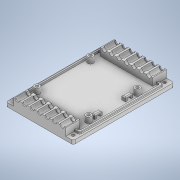
# Autodesk Inventor part: Enclosure Box
Saved by Autodesk Inventor 2021 (Build 250183000, 183)
## iProperties
Created: 2021-06-04
Part Number: Enclosure Box
Material: Generic
Document SubType Name: Modeling
Designer: Anton
Density: 1 g/cm^3
Appearance: Default
Author: Anton
Autodesk Inventor part; units mm, degrees
ref_plane "YZ Plane" through (0, 0, 0) normal (1, 0, 0) x (0, 1, 0)
ref_plane "XZ Plane" through (0, 0, 0) normal (0, 1, 0) x (-1, 0, 0)
ref_plane "XY Plane" through (0, 0, 0) normal (0, 0, 1) x (1, 0, 0)
sketch "Sketch2" plane through (0, 0, 0) normal (0, 1, 0) x (-1, 0, 0)
  line L0 (0, 0) -> (62, 0)
  line L1 (62, 0) -> (62, -66)
  line L2 (62, -66) -> (0, -66)
  line L3 (0, -66) -> (0, 0)
  circle A0 centre (58.15, -9.3) radius 1.5
  circle A1 centre (57.35, -60.86) radius 1.5
  circle A2 centre (3, -4.5) radius 1.5
  circle A3 centre (3, -61.9) radius 1.5
  circle A4 centre (3, -4.5) radius 3
  circle A5 centre (58.15, -9.3) radius 3
  circle A6 centre (57.35, -60.86) radius 3
  circle A7 centre (3, -61.9) radius 3
  line L4 (63, 20) -> (-1, 20)
  line L5 (-1, 20) -> (-1, -86)
  line L6 (-1, -86) -> (63, -86)
  line L7 (63, -86) -> (63, 20)
  dimension "d14" = 66
  dimension "d15" = 62
  dimension "d16" = 3
  dimension "d17" = 3
  dimension "d18" = 3
  dimension "d19" = 3
  dimension "d20" = 3
  dimension "d21" = 4.5
  dimension "d22" = 6
  dimension "d23" = 3
  dimension "d24" = 57.4
  dimension "d25" = 54.35
  dimension "d26" = 0.8
  dimension "d27" = 51.56
  dimension "d28" = 4.8
  dimension "d29" = 6
  dimension "d30" = 6
  dimension "d31" = 6
  dimension "d32" = 20
  dimension "d33" = 20
  dimension "d34" = 1
  dimension "d35" = 1
  constraints: 16 end point, 8 centre point, 4 coincident, 4 parallel, 2 horizontal, 2 perpendicular
  measures "d14" distance between parallel lines of L2 L0
  measures "d15" distance between parallel lines of L3 L1
  measures "d16" diameter of A0
  measures "d17" diameter of A1
  measures "d18" diameter of A3
  measures "d19" diameter of A2
  measures "d20" distance from line of L3 A2.centre
  measures "d21" distance from line of A2.centre L0
  measures "d22" diameter of A4
  measures "d23" distance from line of L3 A3.centre
  measures "d24" distance of A2.centre A3.centre
  measures "d25" horizontal distance of A1.centre A3.centre
  measures "d26" horizontal distance of A1.centre A0.centre
  measures "d27" vertical distance of A1.centre A0.centre
  measures "d28" vertical distance of A2.centre A0.centre
  measures "d29" diameter of A5
  measures "d30" diameter of A6
  measures "d31" diameter of A7
  measures "d32" distance between parallel lines of L4 L0
  measures "d33" distance between parallel lines of L2 L6
  measures "d34" distance between parallel lines of L7 L1
  measures "d35" distance between parallel lines of L3 L5
extrude "Extrusion1" add sketch "Sketch2" along normal blind 2 contours A4 | A7 | L0 L1 L2 L3 | A0 | A1 | A2 | A3 | A5 | A6 | L7 L6 L5 L4
sketch "Sketch4" plane through (0, 2, 0) normal (0, 1, 0) x (1, 0, 0)
  line L0 (-62, 66) -> (0, 66)
  line L1 (0, 66) -> (0, 0)
  line L2 (0, 0) -> (-62, 0)
  line L3 (-62, 0) -> (-62, 66)
  circle A0 centre (-3.85, 56.7) radius 1.5
  circle A1 centre (-4.65, 5.14) radius 1.5
  circle A2 centre (-59, 61.5) radius 1.5
  circle A3 centre (-59, 4.1) radius 1.5
  circle A4 centre (-59, 61.5) radius 3
  circle A5 centre (-3.85, 56.7) radius 3
  circle A6 centre (-4.65, 5.14) radius 3
  circle A7 centre (-59, 4.1) radius 3
  line L4 (1, 86) -> (-63, 86)
  line L5 (-63, 86) -> (-63, -20)
  line L6 (-63, -20) -> (1, -20)
  line L7 (1, -20) -> (1, 86)
  line L8 (1, 86) -> (-63, 86) projected
  line L9 (-63, 86) -> (-63, -20) projected
  point P0 (0, 0)
  dimension "d38" = 66
  dimension "d39" = 62
  dimension "d40" = 3
  dimension "d41" = 3
  dimension "d42" = 3
  dimension "d43" = 3
  dimension "d44" = 3
  dimension "d45" = 4.5
  dimension "d46" = 6
  dimension "d47" = 3
  dimension "d48" = 57.4
  dimension "d49" = 54.35
  dimension "d50" = 0.8
  dimension "d51" = 51.56
  dimension "d52" = 4.8
  dimension "d53" = 6
  dimension "d54" = 6
  dimension "d55" = 6
  dimension "d56" = 20
  dimension "d57" = 20
  dimension "d58" = 1
  dimension "d59" = 1
  dimension "d60" = 0
  dimension "d61" = 0
  constraints: 16 end point, 8 centre point, 4 coincident, 4 parallel, 2 horizontal, 2 perpendicular
  measures "d38" distance between parallel lines of L2 L0
  measures "d39" distance between parallel lines of L3 L1
  measures "d40" diameter of A0
  measures "d41" diameter of A1
  measures "d42" diameter of A3
  measures "d43" diameter of A2
  measures "d44" distance from line of L3 A2.centre
  measures "d45" distance from line of A2.centre L0
  measures "d46" diameter of A4
  measures "d47" distance from line of L3 A3.centre
  measures "d48" distance of A2.centre A3.centre
  measures "d49" horizontal distance of A1.centre A3.centre
  measures "d50" horizontal distance of A1.centre A0.centre
  measures "d51" vertical distance of A1.centre A0.centre
  measures "d52" vertical distance of A2.centre A0.centre
  measures "d53" diameter of A5
  measures "d54" diameter of A6
  measures "d55" diameter of A7
  measures "d56" distance between parallel lines of L4 L0
  measures "d57" distance between parallel lines of L2 L6
  measures "d58" distance between parallel lines of L7 L1
  measures "d59" distance between parallel lines of L3 L5
  measures "d60" distance between parallel lines of L8 L4
  measures "d61" distance between parallel lines of L9 L5
extrude "Extrusion2" add sketch "Sketch4" along normal blind 6 contours A4 | A7 | A5 | A6
sketch "Sketch5" plane through (1, 0, 20) normal (1, 0, 0) x (0, 0, -1)
  line L0 (106, 2) -> (0, 2) projected
  line L1 (36, 2) -> (36, 4)
  line L2 (36, 4) -> (32, 4)
  line L3 (32, 4) -> (32, 2)
  line L4 (69, 2) -> (69, 4)
  line L5 (69, 4) -> (65, 4)
  line L6 (65, 4) -> (65, 2)
  line L7 (71, 2) -> (71, 6)
  line L8 (71, 6) -> (63, 6)
  line L9 (63, 6) -> (63, 2)
  line L10 (38, 2) -> (38, 6)
  line L11 (38, 6) -> (30, 6)
  line L12 (30, 6) -> (30, 2)
  line L13 (30, 2) -> (32, 2)
  line L14 (36, 2) -> (38, 2)
  line L15 (63, 2) -> (65, 2)
  line L16 (69, 2) -> (71, 2)
  line L17 (0, 0) -> (0, 2) projected
  line L18 (106, 0) -> (106, 2) projected
  point P0 (20, 0)
  point P1 (69, 2)
  dimension "d64" = 2
  dimension "d65" = 0
  dimension "d66" = 2
  dimension "d67" = 2
  dimension "d68" = 30
  dimension "d69" = 4
  dimension "d70" = 4
  dimension "d71" = 4
  dimension "d72" = 2
  dimension "d73" = 2
  dimension "d74" = 2
  dimension "d75" = 2
  dimension "d76" = 35
  constraints: 32 end point, 8 parallel, 4 horizontal, 4 perpendicular, 4 point on line
  measures "d64" distance between parallel lines of L11 L2
  measures "d65" distance between parallel lines of L0 L14
  measures "d66" distance between parallel lines of L10 L1
  measures "d67" distance between parallel lines of L12 L3
  measures "d68" distance between parallel lines of L17 L12
  measures "d69" distance between parallel lines of L1 L3
  measures "d70" distance between parallel lines of L0 L11
  measures "d71" distance between parallel lines of L4 L6
  measures "d72" distance between parallel lines of L4 L7
  measures "d73" distance between parallel lines of L9 L6
  measures "d74" distance between parallel lines of L8 L5
  measures "d75" distance between parallel lines of L0 L5
  measures "d76" distance between parallel lines of L18 L7
extrude "Extrusion3" add sketch "Sketch5" against normal blind 8 contours L0 L4 L5 L6 L9 L8 L7 | L0 L1 L2 L3 L12 L11 L10
sketch "Sketch6" plane through (1, 0, 20) normal (1, 0, 0) x (0, 0, -1)
  line L0 (106, 2) -> (0, 2) projected
  line L1 (29.1739, 2) -> (71.7255, 2)
  line L2 (71.7255, 2) -> (71.7255, 7.2821)
  line L3 (71.7255, 7.2821) -> (29.1739, 7.2821)
  line L4 (29.1739, 7.2821) -> (29.1739, 2)
  point P0 (20, 0)
  constraints: 8 end point, 2 parallel, 1 horizontal, 1 perpendicular, 1 point on line
extrude "Extrusion4" cut sketch "Sketch6" against normal blind 4
fillet "Fillet1" radius 1 2 edges at (-5, 4, -45) (-5, 4, -49)
fillet "Fillet2" radius 1 2 edges at (-5, 4, -12) (-5, 4, -16)
fillet "Fillet3" radius 1 8 edges at (-7, 6, -14) (-5, 6, -10) (-3, 6, -14) (-5, 6, -18) (-5, 6, -43) (-3, 6, -47) (-5, 6, -51) (-7, 6, -47)
sketch "Sketch10" plane through (0, 2, 0) normal (0, 1, 0) x (1, 0, 0)
  line L0 (-63, -20) -> (1, -20) projected
  line L1 (-63, 86) -> (-63, -20) projected
  line L2 (1, -20) -> (-63, -20)
  line L3 (-63, -20) -> (-63, -5)
  line L4 (-63, -5) -> (1, -5)
  line L5 (1, -5) -> (1, -20)
  line L6 (1, 86) -> (-63, 86) projected
  line L7 (1, 86) -> (-63, 86)
  line L8 (-63, 86) -> (-63, 71)
  line L9 (-63, 71) -> (1, 71)
  line L10 (1, 71) -> (1, 86)
  line L11 (-59, -20) -> (-3, -20)
  line L12 (-3, -20) -> (-3, -8)
  line L13 (-3, -8) -> (-59, -8)
  line L14 (-59, -8) -> (-59, -20)
  line L15 (-59, 86) -> (-3, 86)
  line L16 (-3, 86) -> (-3, 74)
  line L17 (-3, 74) -> (-59, 74)
  line L18 (-59, 74) -> (-59, 86)
  point P0 (0, 0)
  dimension "d122" = 15
  dimension "d123" = 15
  dimension "d124" = 56
  dimension "d125" = 4
  dimension "d126" = 12
  dimension "d127" = 56
  dimension "d128" = 4
  dimension "d129" = 12
  constraints: 32 end point, 8 parallel, 4 horizontal, 4 perpendicular, 4 point on line
  measures "d122" distance between parallel lines of L9 L6
  measures "d123" distance between parallel lines of L0 L4
  measures "d124" distance between parallel lines of L12 L14
  measures "d125" distance between parallel lines of L1 L14
  measures "d126" distance between parallel lines of L13 L2
  measures "d127" distance between parallel lines of L16 L18
  measures "d128" distance between parallel lines of L1 L18
  measures "d129" distance between parallel lines of L15 L17
extrude "Extrusion7" add sketch "Sketch10" along normal blind 8 contours L14 L13 L12 L0 | L6 L16 L17 L18
sketch "Sketch11" plane through (1, 0, -86) normal (0, 0, -1) x (-1, 0, 0)
  line L0 (60, 10) -> (4, 10) projected
  circle A0 centre (8, 10) radius 3
  line L1 (4, 2) -> (4, 10) projected
  circle A1 centre (16, 10) radius 3
  circle A2 centre (24, 10) radius 3
  circle A3 centre (32, 10) radius 3
  circle A4 centre (40, 10) radius 3
  circle A5 centre (48, 10) radius 3
  circle A6 centre (56, 10) radius 3
  point P0 (1, 0)
  point P1 (29, 10)
  point P2 (35, 10)
  point P3 (21, 10)
  point P4 (27, 10)
  point P5 (5, 10)
  point P6 (11, 10)
  dimension "d132" = 6
  dimension "d133" = 4
  dimension "d136" = 8
  constraints: 7 centre point, 1 horizontal, 1 point on line, 12 other
  measures "d132" diameter of A0
  measures "d133" distance from line of L1 A0.centre
  measures "d136" distance of A0.centre A1.centre
extrude "Extrusion8" cut sketch "Sketch11" against normal blind 11 contours A6 L0 | L0 A6 | A5 L0 | L0 A5 | A4 L0 | L0 A4 | A3 L0 | A2 L0 | A1 L0 | L0 A1 | A0 L0 picked at (31.5599, 8.3609) picked at (23.6454, 9.065) picked at (8.1205, 9.0073)
sketch "Sketch12" plane through (-63, 0, 20) normal (0, 0, 1) x (1, 0, 0)
  line L0 (4, 10) -> (60, 10) projected
  circle A0 centre (56, 10) radius 3.1
  line L1 (60, 2) -> (60, 10) projected
  circle A1 centre (48, 10) radius 3.1
  circle A2 centre (40, 10) radius 3.1
  circle A3 centre (32, 10) radius 3.1
  circle A4 centre (24, 10) radius 3.1
  circle A5 centre (16, 10) radius 3.1
  circle A6 centre (8, 10) radius 3.1
  point P0 (63, 0)
  point P1 (11.1, 10)
  point P2 (4.9, 10)
  point P3 (19.1, 10)
  point P4 (12.9, 10)
  point P5 (27.1, 10)
  point P6 (20.9, 10)
  point P7 (35.1, 10)
  point P8 (28.9, 10)
  point P9 (43.1, 10)
  point P10 (36.9, 10)
  point P11 (51.1, 10)
  point P12 (44.9, 10)
  point P13 (59.1, 10)
  point P14 (52.9, 10)
  dimension "d143" = 6.2
  dimension "d144" = 4
  dimension "d147" = 8
  constraints: 7 centre point, 1 horizontal, 1 point on line, 12 other
  measures "d143" diameter of A0
  measures "d144" distance from line of L1 A0.centre
  measures "d147" distance of A0.centre A1.centre
extrude "Extrusion9" cut sketch "Sketch12" against normal blind 11 contours L0 A6 | L0 A5 | L0 A4 | L0 A3 | L0 A2 | L0 A1 | L0 A0 picked at (6.9967, 9.7527) picked at (15.055, 9.2725) picked at (23.413, 8.1892) picked at (32.945, 9.2725) picked at (39.413, 9.1496) picked at (47.413, 9.1496) picked at (55.413, 9.1496)
sketch "Sketch13" plane through (0, 2, 0) normal (0, 1, 0) x (1, 0, 0)
  line L0 (1, -20) -> (1, 86) projected
  line L1 (1, -20) -> (-63, -20)
  line L2 (-63, -20) -> (-63, -21)
  line L3 (-63, -21) -> (1, -21)
  line L4 (1, -21) -> (1, -20)
  line L5 (1, 86) -> (-63, 86)
  line L6 (-63, 86) -> (-63, 87)
  line L7 (-63, 87) -> (1, 87)
  line L8 (1, 87) -> (1, 86)
  point P0 (-63, -20)
  dimension "d158" = 1
  dimension "d159" = 1
  constraints: 16 end point, 4 parallel, 2 horizontal, 2 perpendicular, 1 point on line
  measures "d158" distance of L5.end L6.end
  measures "d159" distance of L1.end L2.end
extrude "Extrusion10" add sketch "Sketch13" along normal blind 8 and the other way blind 2
sketch "Sketch14" plane through (0, 2, 0) normal (0, 1, 0) x (1, 0, 0)
  line L0 (-63, 87) -> (1, 87) projected
  line L1 (-63, 87) -> (-67, 87)
  line L2 (-67, 87) -> (-67, -21)
  line L3 (-67, -21) -> (-63, -21)
  line L4 (-63, -21) -> (-63, 87)
  line L5 (1, -21) -> (1, 87) projected
  line L6 (1, -21) -> (5, -21)
  line L7 (5, -21) -> (5, 87)
  line L8 (5, 87) -> (1, 87)
  line L9 (1, 87) -> (1, -21)
  line L10 (-63, -21) -> (1, -21) projected
  point P0 (0, 0)
  dimension "d164" = 0
  dimension "d165" = 4
  dimension "d166" = 4
  dimension "d167" = 0
  constraints: 16 end point, 4 parallel, 2 horizontal, 2 perpendicular
  measures "d164" distance between parallel lines of L10 L3
  measures "d165" distance between parallel lines of L2 L4
  measures "d166" distance between parallel lines of L5 L7
  measures "d167" distance between parallel lines of L0 L8
extrude "Extrusion11" add sketch "Sketch14" against normal blind 2 contours L4 L3 L2 L1 | L8 L7 L6 L5
sketch "Sketch16" plane through (0, 2, 0) normal (0, 1, 0) x (1, 0, 0)
  line L0 (-3, -20) -> (-3, -8) projected
  line L1 (-3, -8) -> (-59, -8)
  line L2 (-59, -8) -> (-59, -6)
  line L3 (-59, -6) -> (-3, -6)
  line L4 (-3, -6) -> (-3, -8)
  line L5 (-3, 74) -> (-3, 86) projected
  line L6 (-3, 74) -> (-59, 74)
  line L7 (-59, 74) -> (-59, 72)
  line L8 (-59, 72) -> (-3, 72)
  line L9 (-3, 72) -> (-3, 74)
  point P0 (0, 0)
  dimension "d177" = 2
  dimension "d178" = 2
  constraints: 16 end point, 4 parallel, 2 horizontal, 2 perpendicular
  measures "d177" distance between parallel lines of L8 L6
  measures "d178" distance between parallel lines of L1 L3
extrude "Extrusion12" add sketch "Sketch16" along normal blind 8
sketch "Sketch17" plane through (0, 2, 0) normal (0, 1, 0) x (1, 0, 0)
  line L0 (-58, 78) -> (-63, 78)
  line L1 (-58, -12) -> (-63, -12)
  line L2 (-4, -12) -> (1, -12)
  line L3 (-65, 76) -> (-65, -10)
  line L4 (-4, 78) -> (1, 78)
  line L5 (3, -10) -> (3, 76)
  arc A0 (-65, -10) -> (-63, -12) centre (-63, -10) ccw
  arc A1 (-63, 78) -> (-65, 76) centre (-63, 76) ccw
  arc A2 (1, -12) -> (3, -10) centre (1, -10) ccw
  arc A3 (3, 76) -> (1, 78) centre (1, 76) ccw
  line L6 (-56, -10) -> (-61, -10)
  line L7 (-63, -8) -> (-63, 74)
  line L8 (-61, 76) -> (-56, 76)
  line L9 (-6, 76) -> (-1, 76)
  line L10 (1, 74) -> (1, -8)
  line L11 (-1, -10) -> (-6, -10)
  arc A4 (-1, -10) -> (1, -8) centre (-1, -8) ccw
  arc A5 (1, 74) -> (-1, 76) centre (-1, 74) ccw
  arc A6 (-63, -8) -> (-61, -10) centre (-61, -8) ccw
  arc A7 (-61, 76) -> (-63, 74) centre (-61, 74) ccw
  line L12 (-3, -20) -> (-3, -6) projected
  line L13 (-3, -10) -> (-3, -12)
  line L14 (-3, 72) -> (-3, 86) projected
  line L15 (-3, 76) -> (-3, 78)
  line L16 (-59, -6) -> (-59, -20) projected
  line L17 (-59, -12) -> (-59, -10)
  line L18 (-59, 86) -> (-59, 72) projected
  line L19 (-59, 76) -> (-59, 78)
  point P0 (0, 0)
  point P1 (-67, -21)
  point P2 (-67, 87)
  point P3 (5, -21)
  point P4 (5, 87)
  dimension "d199" = 2
  dimension "d200" = 2
  dimension "d201" = 2
  dimension "d202" = 2
  constraints: 32 end point, 17 point on line, 16 point on circle, 16 tangent, 8 centre point, 6 equal radius, 1 parallel, 4 other
  measures "d199" radius of A0
  measures "d200" distance between parallel lines of L3 L7
  measures "d201" distance between parallel lines of L5 L10
  measures "d202" radius of A4
extrude "Extrusion13" add sketch "Sketch17" along normal blind 2
fillet "Fillet8" radius 0.5 5 edges at (2.4142, 4, -77.4142) (-1, 4, -78) (2.4142, 4, 11.4142) (-1, 4, 12) (3, 4, -33)
fillet "Fillet9" radius 0.5 5 edges at (-65, 4, -33) (-64.4142, 4, 11.4142) (-61, 4, 12) (-64.4142, 4, -77.4142) (-61, 4, -78)
sketch "Sketch19" plane through (0, 2, 0) normal (0, 1, 0) x (1, 0, 0)
  line L0 (-3, -12) -> (-3, -20) projected
  line L1 (-3, -19.2005) -> (2.1145, -19.2005)
  line L2 (2.1145, -19.2005) -> (2.1145, -23.3897)
  line L3 (2.1145, -23.3897) -> (-3, -23.3897)
  line L4 (-3, -23.3897) -> (-3, -19.2005)
  line L5 (-59, -6) -> (-59, -20) projected
  line L6 (-59, -18.8883) -> (-64.246, -18.8883)
  line L7 (-64.246, -18.8883) -> (-64.246, -22.9002)
  line L8 (-64.246, -22.9002) -> (-59, -22.9002)
  line L9 (-59, -22.9002) -> (-59, -18.8883)
  line L10 (-3, 72) -> (-3, 86) projected
  line L11 (-3, 84.9198) -> (1.5867, 84.9198)
  line L12 (1.5867, 84.9198) -> (1.5867, 89.8515)
  line L13 (1.5867, 89.8515) -> (-3, 89.8515)
  line L14 (-3, 89.8515) -> (-3, 84.9198)
  line L15 (-59, 78) -> (-59, 86) projected
  line L16 (-59, 82.7172) -> (-64.4827, 82.7172)
  line L17 (-64.4827, 82.7172) -> (-64.4827, 89.8515)
  line L18 (-64.4827, 89.8515) -> (-59, 89.8515)
  line L19 (-59, 89.8515) -> (-59, 82.7172)
  point P0 (0, 0)
  constraints: 32 end point, 8 parallel, 5 point on line, 4 horizontal, 4 perpendicular
extrude "Extrusion14" cut sketch "Sketch19" along normal blind 10
sketch "Sketch20" plane through (0, 0, 0) normal (0, -1, 0) x (1, 0, 0)
  line L0 (5, 21) -> (-67, 21) projected
  line L1 (-67, -87) -> (-67, 21) projected
  line L2 (5, 21) -> (-67, 21)
  line L3 (-67, 21) -> (-67, -87)
  line L4 (-67, -87) -> (5, -87)
  line L5 (5, -87) -> (5, 21)
  point P0 (0, 0)
  constraints: 8 end point, 2 parallel, 1 horizontal, 1 perpendicular
extrude "Extrusion15" add sketch "Sketch20" along normal blind 2
sketch "Sketch21" plane through (0, 2, 0) normal (0, 1, 0) x (1, 0, 0)
  circle A0 centre (0, -16) radius 4
  line L0 (-3, -21) -> (5, -21) projected
  line L1 (5, -21) -> (5, 87) projected
  circle A1 centre (0, -16) radius 1.5
  circle A2 centre (-62, -16) radius 4
  circle A3 centre (-62, 82) radius 4
  circle A4 centre (0, 82) radius 4
  line L2 (-59, -21) -> (-67, -21) projected
  line L3 (-67, 87) -> (-67, -21) projected
  line L4 (-59, 87) -> (-67, 87) projected
  circle A5 centre (0, 82) radius 1.5
  circle A6 centre (-62, 82) radius 1.5
  circle A7 centre (-62, -16) radius 1.5
  line L5 (-3, 87) -> (5, 87) projected
  point P0 (0, 0)
  dimension "d215" = 8
  dimension "d216" = 5
  dimension "d217" = 5
  dimension "d218" = 3
  dimension "d219" = 8
  dimension "d220" = 8
  dimension "d221" = 8
  dimension "d222" = 5
  dimension "d223" = 5
  dimension "d224" = 5
  dimension "d225" = 5
  dimension "d226" = 3
  dimension "d227" = 3
  dimension "d228" = 3
  dimension "d260" = 5
  dimension "d261" = 5
  constraints: 8 centre point, 4 coincident
  measures "d215" diameter of A0
  measures "d216" distance from line of L0 A0.centre
  measures "d217" distance from line of L1 A0.centre
  measures "d218" diameter of A1
  measures "d219" diameter of A2
  measures "d220" diameter of A3
  measures "d221" diameter of A4
  measures "d222" distance from line of L2 A2.centre
  measures "d223" distance from line of L3 A2.centre
  measures "d224" distance from line of L3 A3.centre
  measures "d225" distance from line of L4 A3.centre
  measures "d226" diameter of A7
  measures "d227" diameter of A6
  measures "d228" diameter of A5
  measures "d260" distance from line of L1 A4.centre
  measures "d261" distance from line of L5 A5.centre
extrude "Extrusion16" cut sketch "Sketch21" against normal mid plane 10 contours A1 | A5 | A6 | A7
sketch "Sketch22" plane through (0, -2, 0) normal (0, -1, 0) x (1, 0, 0)
  circle A0 centre (0, 16) radius 1.5 projected
  circle A1 centre (0, 16) radius 3.5
  circle A2 centre (-62, 16) radius 1.5 projected
  circle A3 centre (-62, 16) radius 3.5
  circle A4 centre (-62, -82) radius 1.5 projected
  circle A5 centre (0, -82) radius 1.5 projected
  circle A6 centre (0, -82) radius 3.5
  circle A7 centre (-62, -82) radius 3.5
  point P0 (0, 0)
  point P1 (-63, -78)
  dimension "d231" = 7
  dimension "d232" = 7
  dimension "d233" = 7
  dimension "d234" = 7
  constraints: 4 centre point, 4 coincident
  measures "d231" diameter of A6
  measures "d232" diameter of A1
  measures "d233" diameter of A3
  measures "d234" diameter of A7
extrude "Extrusion17" cut sketch "Sketch22" against normal blind 2
fillet "Fillet11" radius 2 4 edges at (5, 0, -87) (-67, 0, -87) (-67, 0, 21) (5, 0, 21)
sketch "Sketch23" plane through (-59, 10, 21) normal (0, 0, 1) x (1, 0, 0)
  line L0 (56, 0) -> (0, 0) projected
  circle A0 centre (4, 0) radius 2.25
  circle A1 centre (12, 0) radius 2.25
  circle A2 centre (20, 0) radius 2.25
  circle A3 centre (28, 0) radius 2.25
  circle A4 centre (36, 0) radius 2.25
  circle A5 centre (44, 0) radius 2.25
  circle A6 centre (52, 0) radius 2.25
  point P0 (59, -10)
  point P1 (49.75, 0)
  point P2 (54.25, 0)
  point P3 (41.75, 0)
  point P4 (46.25, 0)
  point P5 (33.75, 0)
  point P6 (38.25, 0)
  point P7 (17.75, 0)
  point P8 (22.25, 0)
  point P9 (9.75, 0)
  point P10 (14.25, 0)
  point P11 (1.75, 0)
  point P12 (6.25, 0)
  dimension "d238" = 4.5
  dimension "d239" = 4
  dimension "d242" = 8
  constraints: 7 centre point, 1 horizontal, 1 point on line, 12 other
  measures "d238" diameter of A0
  measures "d239" distance of L0.end A0.centre
  measures "d242" distance of A0.centre A1.centre
extrude "Extrusion18" cut sketch "Sketch23" against normal blind 20 contours A6 L0 | A5 L0 | A4 L0 | A3 L0 | L0 A3 | A2 L0 | A1 L0 | A0 L0 picked at (51.9096, -0.7445) picked at (43.9096, -0.7445) picked at (35.9096, -0.7445) picked at (19.9096, -0.7445) picked at (11.4604, -0.6768) picked at (3.9955, -1.0931)
sketch "Sketch24" plane through (-3, 10, -87) normal (0, 0, -1) x (-1, 0, 0)
  line L0 (56, 0) -> (0, 0) projected
  circle A0 centre (4, 0) radius 2.25
  line L1 (0, 0) -> (0, -8) projected
  circle A1 centre (12, 0) radius 2.25
  circle A2 centre (20, 0) radius 2.25
  circle A3 centre (28, 0) radius 2.25
  circle A4 centre (36, 0) radius 2.25
  circle A5 centre (44, 0) radius 2.25
  circle A6 centre (52, 0) radius 2.25
  point P0 (-3, -10)
  point P1 (1.75, 0)
  point P2 (6.25, 0)
  point P3 (9.75, 0)
  point P4 (14.25, 0)
  point P5 (17.75, 0)
  point P6 (22.25, 0)
  point P7 (25.75, 0)
  point P8 (30.25, 0)
  point P9 (33.75, 0)
  point P10 (38.25, 0)
  point P11 (49.75, 0)
  point P12 (54.25, 0)
  dimension "d249" = 4
  dimension "d250" = 4.5
  dimension "d253" = 8
  constraints: 7 centre point, 1 horizontal, 1 point on line, 12 other
  measures "d249" distance from line of L1 A0.centre
  measures "d250" diameter of A0
  measures "d253" distance of A0.centre A1.centre
extrude "Extrusion19" cut sketch "Sketch24" against normal blind 20 contours A6 L0 | A5 L0 | L0 A5 | A4 L0 | A3 L0 | A2 L0 | A1 L0 | A0 L0 picked at (51.9096, -0.7445) picked at (35.9096, -0.7445) picked at (27.9096, -0.7445) picked at (19.9096, -0.7445) picked at (11.4604, -0.6768) picked at (3.9955, -1.0931)
body "Solid1"
